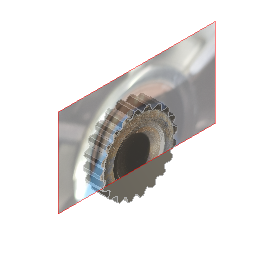
test spline 37.5 v1 (Autodesk Fusion 360 design; units mm, degrees)
Autodesk Fusion 360 part; units mm, degrees
sketch "Sketch1" plane through (0, 0, 0) normal (1, 0, 0) x (0, 1, 0)
  circle A0 centre (0, 0) radius 10.5508 construction
  line L0 (0, 0) -> (0, -4.2525) construction
  line L1 (-1.4567, 11.2085) -> (0, 9.5926)
  line L2 (0, 9.5926) -> (1.4593, 11.2114)
  arc A1 (3.7927, 9.0309) -> (-2.1823, 9.5488) centre (0, 0) ccw
  arc A2 (4.1612, 9.1645) -> (-2.8648, 9.6487) centre (0, 0) ccw
  line L3 (0.0124, -0.0021) -> (0.834, 10.5178) construction
  line L4 (0, 0) -> (-0.834, 10.5178) construction
  line L5 (0.834, 10.5178) -> (0.4107, 10.8994) construction
  line L6 (-0.834, 10.5178) -> (-0.4545, 10.8599) construction
  line L7 (0.834, 10.5178) -> (0.3009, 10.5601) construction
  line L8 (-0.834, 10.5178) -> (-0.4013, 10.5521) construction
  circle A3 centre (0, 0) radius 11.0365
  circle A4 centre (-0.1167, 9.9409) radius 0.1466
  circle A5 centre (0.1167, 9.9409) radius 0.1466
  circle A6 centre (0.0124, -0.0021) radius 11.3065
  circle A7 centre (-1.5138, 11.053) radius 0.1466
  circle A8 centre (1.5166, 11.056) radius 0.1466
  line L9 (0, 9.5926) -> (0, 12.8891) construction
  dimension "d1" = 21.1016
  dimension "d8" = 9.795
  dimension "d9" = 10.065
  dimension "d26" = 9
  dimension "d28" = 37.5
  dimension "d29" = 37.5
  dimension "d32" = 22.073
  dimension "d36" = 0.2931
  dimension "d37" = 22.613
  dimension "d38" = 84.068
  constraint coincident A0.centre L0.start
  constraint vertical L0
  constraint coincident A0 L4.end
  constraint coincident A0 L3.end
  constraint symmetric L0 L3.end L4.end
  constraint coincident L2 L3.end
  constraint coincident L1 L4.end
  constraint coincident L1.end L2.start
  constraint coincident L0 L1.end
  constraint perpendicular L2 L5
  constraint perpendicular L1 L6
  constraint tangent A0 L8
  constraint tangent A0 L7
  constraint equal A4 A5
  constraint tangent A1 A4
  constraint tangent L1 A4
  constraint tangent A1 A5
  constraint tangent L2 A5
  constraint coincident L3.start A6.centre
  constraint coincident L2.end A6
  constraint coincident L1.start A6
  constraint equal A4 A8
  constraint equal A4 A7
  constraint tangent A6 A7
  constraint tangent L1 A7
  constraint tangent L2 A8
  constraint tangent A6 A8
  constraint vertical L9
  measures "d1" diameter of A0
  measures "d8" radius of A1
  measures "d9" radius of A2
  measures "d26" angle of L3 L4
  measures "d28" angle of L5 L7
  measures "d29" angle of L6 L8
  measures "d32" diameter of A3
  measures "d36" diameter of A4
  measures "d37" diameter of A6
  measures "d38" angle of L1 L2
sketch "Sketch2" plane through (0, 0, 0) normal (1, 0, 0) x (0, 1, 0)
  circle A0 centre (0, 0) radius 11.0365
  arc A1 (3.7927, 9.0309) -> (-2.1823, 9.5488) centre (0, 0) ccw
  line L0 (0, 9.5926) -> (1.4593, 11.2114)
  line L1 (-1.4567, 11.2085) -> (0, 9.5926)
  dimension "d31" = 22.073
  constraint coincident A0.centre A1.centre
  measures "d31" diameter of A0
extrude "Extrude1" add sketch "Sketch1" sketch "Sketch2" along normal blind 5 contours L1 A1 A4 | L1 L2 A1 | L2 A1 A5 of sketch 2 contours A0 L0 L1
pattern_circular "C-Pattern1" count 20 over 360 about axis through (1.75, 0, 0) along (1, 0, 0) of 5 faces at (1.6667, -0.901, 10.5921) (1.6667, 0.0894, 9.7946) (3.3333, -0.1287, 9.7948) (1.6667, 0.1218, 9.7944) (1.6667, 0.5633, 10.2174)
move_body "Move1" bodies 1 to x (1, 0, 0) y (0, 1, 0) z (0, 0, 1) at (0, 1.5, -5.5)
move_body "Move2" bodies 1 to x (1, 0, 0) y (0, 0.996195, -0.087156) z (0, 0.087156, 0.996195) at (0, 0.4851, 0.1098)
equation "modulus = 0.977 mm" comment "modulus"
equation "D2 = 21.5864825 mm" comment "Diameter modulus"
equation "d36 = modulus * 0.3"
